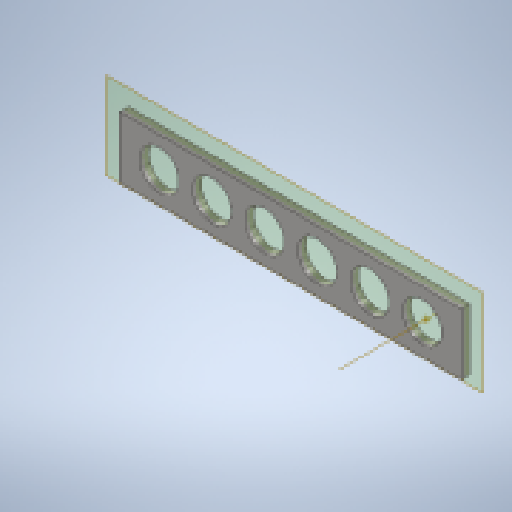
# Autodesk Inventor part: Ball_Spacers
Saved by Autodesk Inventor 2025.2 (Build 292293000, 293)
## iProperties
Created: 2024-12-11
Part Number: Ball_Spacers
Material: Steel, Carbon
Document SubType Name: Modeling
Designer: konch
Density: 7.85 g/cm^3
Appearance: Semi-Polished
Author: konch
Autodesk Inventor part; units mm, degrees
ref_plane "YZ Plane" through (0, 0, 0) normal (1, 0, 0) x (0, 1, 0)
ref_plane "XZ Plane" through (0, 0, 0) normal (0, 1, 0) x (-1, 0, 0)
ref_plane "XY Plane" through (0, 0, 0) normal (0, 0, 1) x (1, 0, 0)
sketch "Sketch1" plane through (0, 0, 0) normal (0, 0, 1) x (1, 0, 0)
  line L0 (0, 0) -> (39, 0)
  line L1 (39, 0) -> (39, 7)
  line L2 (39, 7) -> (0, 7)
  line L3 (0, 7) -> (0, 0)
  line L4 (39, 3.5) -> (0, 3.5) construction
  line L5 (39, 0) -> (35.662, 0)
  line L6 (39, 3.5) -> (34.5, 3.5) construction
  circle A0 centre (34.5, 3.5) radius 2.25
  line L7 (34.5, 3.5) -> (28.5, 3.5) construction
  circle A1 centre (28.5, 3.5) radius 2.25
  line L8 (28.5, 3.5) -> (22.5, 3.5) construction
  line L9 (22.5, 3.5) -> (16.5, 3.5) construction
  line L10 (16.5, 3.5) -> (10.5, 3.5) construction
  line L11 (10.5, 3.5) -> (4.5, 3.5) construction
  circle A2 centre (22.5, 3.5) radius 2.25
  circle A3 centre (16.5, 3.5) radius 2.25
  circle A4 centre (10.5, 3.5) radius 2.25
  circle A5 centre (4.5, 3.5) radius 2.25
  dimension "d0" = 39
  dimension "d1" = 7
  dimension "d2" = 4.5
  dimension "d3" = 6
  dimension "d4" = 4.5
  dimension "d5" = 6
  dimension "d6" = 6
  dimension "d7" = 6
  dimension "d8" = 6
  dimension "d9" = 4.5
  dimension "d10" = 4.5
  dimension "d11" = 4.5
  dimension "d12" = 4.5
  constraints: 24 end point, 7 point on line, 6 centre point, 6 coincident, 3 perpendicular, 2 midpoint, 1 horizontal
  measures "d0" distance of L0.start L0.end
  measures "d1" distance of L0.end L1.end
  measures "d2" distance of L4.start L6.end
  measures "d3" distance of L7.start L7.end
  measures "d4" diameter of A1
  measures "d5" distance of L8.start L8.end
  measures "d6" distance of L8.end L9.end
  measures "d7" distance of L9.end L10.end
  measures "d8" distance of L10.end L11.end
  measures "d9" diameter of A2
  measures "d10" diameter of A3
  measures "d11" diameter of A4
  measures "d12" diameter of A5
extrude "Extrusion1" add sketch "Sketch1" along normal blind 1
ref_plane "Work Plane1" through (0, 0, 0.6) normal (0, 0, -1) x (-1, 0, 0)
body "Solid1"
